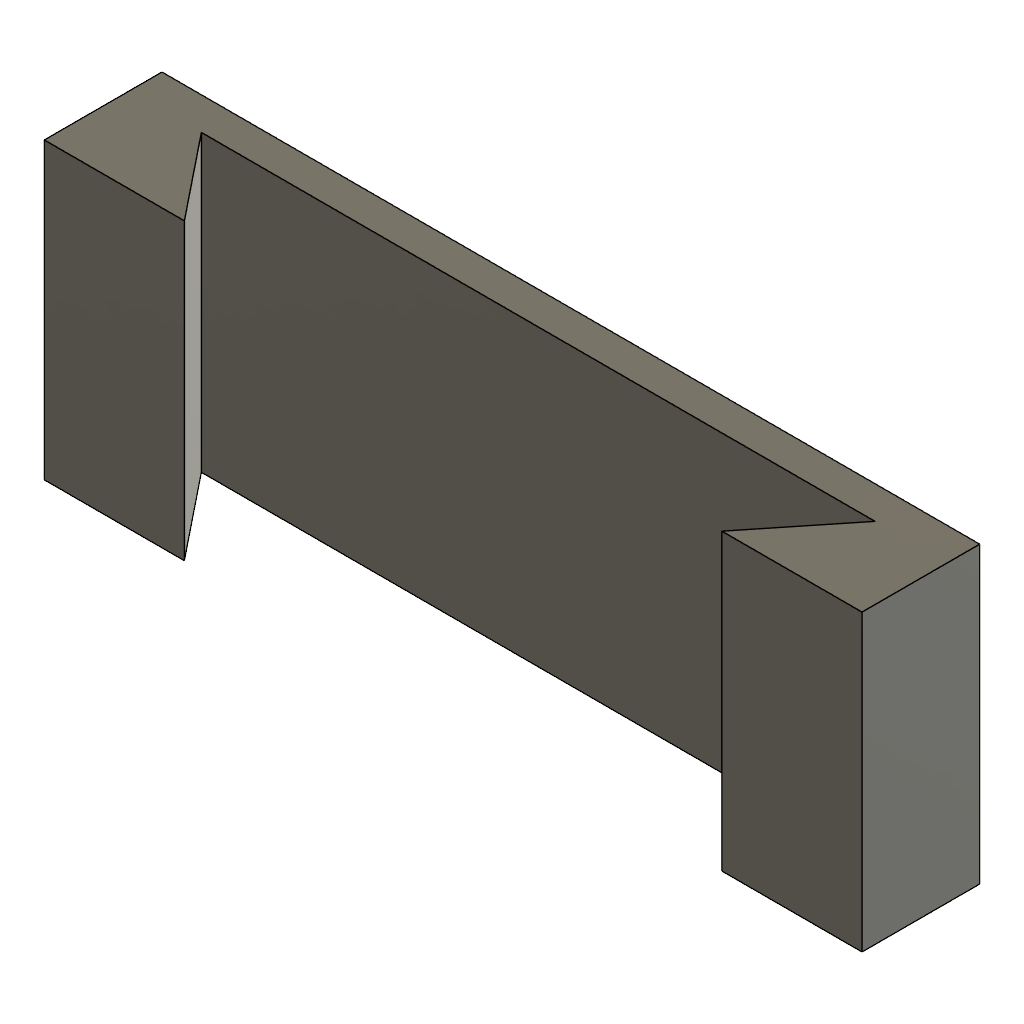
fit_coupon_gap_0.35 (Autodesk Fusion 360 design; units mm, degrees)
part number: 2026-10-03-13-54-33-677
Autodesk Fusion 360 part; units mm, degrees
ref_plane "工作平面1" through (0, 0, 0) normal (0, 0, 1) x (1, 0, 0)
sketch "草图1" plane through (0, 0, 0) normal (0, 0, 1) x (1, 0, 0)
  line L0 (-25, -9) -> (25, -9)
  line L1 (25, -9) -> (25, 9)
  line L2 (25, 9) -> (-25, 9)
  line L3 (-25, 9) -> (-25, -9)
extrude "Coupon base" add sketch "草图1" along normal blind 2
ref_plane "工作平面2" through (0, 0, 2) normal (0, 0, 1) x (1, 0, 0)
sketch "草图2" plane through (0, 0, 2) normal (0, 0, 1) x (1, 0, 0)
  line L0 (-25, -9) -> (-20.59, -9)
  line L1 (-20.59, -9) -> (-20.59, 9)
  line L2 (-20.59, 9) -> (-25, 9)
  line L3 (-25, 9) -> (-25, -9)
ref_plane "工作平面3" through (0, 0, 7.2) normal (0, 0, 1) x (1, 0, 0)
sketch "草图3" plane through (0, 0, 7.2) normal (0, 0, 1) x (1, 0, 0)
  line L0 (-25, -9) -> (-16.43, -9)
  line L1 (-16.43, -9) -> (-16.43, 9)
  line L2 (-16.43, 9) -> (-25, 9)
  line L3 (-25, 9) -> (-25, -9)
loft "Coupon dovetail rail" add profiles "草图2", "草图3" section 1 section 2
ref_plane "工作平面4" through (0, 0, 2) normal (0, 0, 1) x (1, 0, 0)
sketch "草图4" plane through (0, 0, 2) normal (0, 0, 1) x (1, 0, 0)
  line L0 (20.59, -9) -> (25, -9)
  line L1 (25, -9) -> (25, 9)
  line L2 (25, 9) -> (20.59, 9)
  line L3 (20.59, 9) -> (20.59, -9)
ref_plane "工作平面5" through (0, 0, 7.2) normal (0, 0, 1) x (1, 0, 0)
sketch "草图5" plane through (0, 0, 7.2) normal (0, 0, 1) x (1, 0, 0)
  line L0 (16.43, -9) -> (25, -9)
  line L1 (25, -9) -> (25, 9)
  line L2 (25, 9) -> (16.43, 9)
  line L3 (16.43, 9) -> (16.43, -9)
loft "Coupon dovetail rail (1)" add profiles "草图4", "草图5" section 1 section 2
